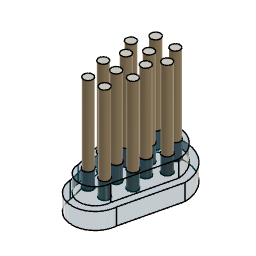
Molde Interior (Autodesk Fusion 360 design; units mm, degrees)
Autodesk Fusion 360 part; units mm, degrees
sketch "Boceto1" plane through (0, 0, 0) normal (0, 0, 1) x (1, 0, 0)
  line L0 (0, 0) -> (0, 9) construction
  arc A0 (-10, 9) -> (10, 9) centre (0, 10.0556) ccw construction
  line L1 (10, 9) -> (14, 26) construction
  arc A1 (14.9995, 25.882) -> (-14.9995, 25.882) centre (0, 26) ccw construction
  line L2 (-10, 9) -> (-14, 26) construction
  line L3 (-10, 9) -> (10, 9) construction
  line L4 (0, 40) -> (0, 26) construction
  arc A2 (-10.9875, 8.8309) -> (10.9875, 8.8309) centre (0, 10.0556) ccw construction
  line L5 (10.9875, 8.8309) -> (14.9995, 25.882) construction
  line L6 (-10.9875, 8.8309) -> (-14.9995, 25.882) construction
  arc A3 (14, 26) -> (-14, 26) centre (0, 26) ccw construction
  line L7 (-14, 26) -> (14, 26) construction
  line L8 (0, 0) -> (0, 40) construction
  arc A4 (10.9951, 26.3275) -> (-10.9951, 26.3275) centre (0, 26) ccw
  line L9 (-7.0326, 9.4867) -> (-10.9951, 26.3275)
  arc A5 (-7.0326, 9.4867) -> (7.0326, 9.4867) centre (0, 10.0556) ccw
  line L10 (7.0326, 9.4867) -> (10.9951, 26.3275)
  dimension "d1" = 1
  dimension "d2" = 40
  dimension "d3" = 9
  dimension "d4" = 14
  dimension "d5" = 28
  dimension "d6" = 20
  dimension "d7" = 3
  constraint coincident L0.start L8.start
  constraint vertical L8
  constraint parallel L0 L8
  constraint parallel L4 L8
  constraint perpendicular L4 L7
  constraint midpoint A1.centre L7
  constraint horizontal L3
  constraint midpoint L0.end L3
  constraint coincident L4.start A3
  constraint coincident L0.start A0
  measures "d2" distance of L0.start L4.start
  measures "d3" distance of L0.end L0.start
  measures "d4" distance of L4.start A1.centre
  measures "d5" distance of L1.end L2.end
  measures "d6" distance of A0.start A0.end
extrude "Extruir1" add sketch "Boceto1" along normal blind 5 makes body 1
sketch "Boceto2" plane through (0, 0, 5) normal (0, 0, 1) x (-1, 0, 0)
  arc A0 (7.0326, -9.4867) -> (-7.0326, -9.4867) centre (0, -10.0556) ccw
  line L0 (-7.0326, -9.4867) -> (-10.9951, -26.3275)
  arc A1 (-10.9951, -26.3275) -> (10.9951, -26.3275) centre (0, -26) ccw
  line L1 (10.9951, -26.3275) -> (7.0326, -9.4867)
  line L2 (8.8845, -26.5258) -> (4.949, -9.8)
  arc A2 (4.949, -9.8) -> (-4.949, -9.8) centre (0, -10.0556) ccw
  line L3 (-4.949, -9.8) -> (-8.8845, -26.5258)
  arc A3 (-8.8845, -26.5258) -> (8.8845, -26.5258) centre (0, -26) ccw
  dimension "d10" = -2.1
extrude "Extruir2" add sketch "Boceto2" along normal blind 5 contours L2 A2 L3 A3 bodies 1
sketch "Boceto3" plane through (0, 0, 10) normal (0, 0, 1) x (-1, 0, 0)
  arc A0 (-8.8845, -26.5258) -> (8.8845, -26.5258) centre (0, -26) ccw
  line L0 (8.8845, -26.5258) -> (4.949, -9.8)
  arc A1 (4.949, -9.8) -> (-4.949, -9.8) centre (0, -10.0556) ccw
  line L1 (-4.949, -9.8) -> (-8.8845, -26.5258)
  line L2 (0, -34.9) -> (0, -5.1) construction
  line L3 (0, -20) -> (7.349, -20) construction
  line L4 (0, -20) -> (-7.349, -20) construction
  circle A2 centre (3, -31.4) radius 1.5
  line L5 (0, -34.9) -> (0, -31.4) construction
  line L6 (0, -31.4) -> (3, -31.4) construction
  circle A3 centre (-3, -31.4) radius 1.5
  line L7 (0, -34.9) -> (0, -26.4) construction
  line L8 (0, -26.4) -> (5.5, -26.4) construction
  circle A4 centre (5.5, -26.4) radius 1.5
  circle A5 centre (-5.5, -26.4) radius 1.5
  circle A6 centre (0, -26.4) radius 1.5
  circle A7 centre (3, -22.4) radius 1.5
  circle A8 centre (-3, -22.4) radius 1.5
  circle A9 centre (0, -16.4) radius 1.5
  circle A10 centre (-3, -10.4) radius 1.5 construction
  circle A11 centre (3, -10.4) radius 1.5 construction
  circle A12 centre (5.5, -17) radius 1.5 construction
  circle A13 centre (-5.5, -17) radius 1.5 construction
  line L9 (5.5, -17) -> (4.5, -17) construction
  circle A14 centre (4.5, -17) radius 1.5
  line L10 (-5.5, -17) -> (-4.5, -17) construction
  circle A15 centre (-4.5, -17) radius 1.5
  line L11 (3, -10.4) -> (2.5, -10.4) construction
  line L12 (-3, -10.4) -> (-2.5, -10.4) construction
  circle A16 centre (2.5, -10.4) radius 1.5
  circle A17 centre (-2.5, -10.4) radius 1.5
  dimension "d13" = 3
  dimension "d14" = 3.5
  dimension "d15" = 3
  dimension "d16" = 3
  dimension "d17" = 3
  dimension "d18" = 5
  dimension "d21" = 0
  dimension "d22" = 9
  dimension "d25" = 0
  dimension "d26" = 10
  dimension "d29" = 0
  dimension "d30" = 21
  dimension "d35" = 5.5
  dimension "d38" = 1
  dimension "d39" = 3
  dimension "d40" = 3
  dimension "d41" = 0.5
  dimension "d42" = 0.5
  dimension "d43" = 3
  dimension "d44" = 3
  dimension "d45" = 1
  constraint midpoint A0 L2.start
  constraint midpoint A1 L2.end
  constraint midpoint L2 L3.start
  constraint coincident L0 L3.end
  constraint perpendicular L2 L3
  constraint coincident L1 L4.end
  constraint perpendicular L2 L4
  constraint parallel L2 L5
  constraint perpendicular L5 L6
  constraint symmetric L2 A2 A3
  constraint coincident L2 L7.end
  constraint parallel L2 L7
  constraint perpendicular L7 L8
  constraint coincident L8.end A4.centre
  constraint symmetric L2 A4 A5
  constraint coincident L7.end L8.start
  constraint coincident A2.centre L6.end
  constraint coincident A12.centre L9.start
  constraint perpendicular L2 L9
  constraint coincident L9.end A14.centre
  constraint coincident A13.centre L10.start
  constraint horizontal L10
  constraint coincident L10.end A15.centre
  constraint coincident A11.centre L11.start
  constraint perpendicular L2 L11
  constraint coincident A10.centre L12.start
  constraint horizontal L12
  constraint coincident L11.end A16.centre
  constraint coincident L12.end A17.centre
  measures "d13" diameter of A2
  measures "d14" distance of L2.start L5.end
  measures "d15" distance of L5.end A2.centre
  measures "d16" diameter of A4
  measures "d17" diameter of A6
  measures "d18" distance of L5.end L7.end
  measures "d35" distance of L7.end L8.end
  measures "d38" distance of A12.centre L9.end
  measures "d39" diameter of A14
  measures "d40" diameter of A15
  measures "d41" distance of A10.centre L12.end
  measures "d42" distance of A11.centre L11.end
  measures "d43" diameter of A16
  measures "d44" diameter of A17
  measures "d45" distance of A13.centre L10.end
extrude "Extruir3" add sketch "Boceto3" along normal blind 24 separate body contours A2 | A3 | A4 | A5 | A6 | A7 | A8 | A9 | A14 | A15 | A16 | A17 makes body 2 at (3.0019, 17.0748, 26) makes body 3 at (4.0019, 26.4748, 26) makes body 4 at (1.5019, 22.4748, 26) makes body 5 at (-4.4981, 22.4748, 26) makes body 6 at (4.4095, 31.913, 26) makes body 7 at (-3.9981, 10.4748, 26) makes body 8 at (-5.9981, 17.0748, 26) makes body 9 at (-6.9981, 26.4748, 26) makes body 10 at (-1.4981, 16.4748, 26) makes body 11 at (-1.4981, 26.4748, 26) makes body 12 at (-1.5905, 31.913, 26) makes body 13 at (1.0019, 10.4748, 26)
extrude "Extruir4" cut sketch "Boceto3" against normal blind 5 contours A2 | A3 | A4 | A5 | A6 | A7 | A8 | A9 | A14 | A15 | A16 | A17 bodies 1
extrude "Extruir5" add 12 faces at (-2.084, 10.2947, 10) (-2.75, 23.2669, 10) (-4.2334, 15.9775, 10) (-0.4671, 16.6898, 10) (2.6931, 10.7148, 10) (4.0495, 16.9321, 10) (3.25, 23.2669, 10) (0.25, 27.2669, 10) (-5.9944, 27.1547, 10) (-2.7722, 31.9804, 10) (3.1605, 32.0128, 10) (5.0329, 26.6898, 10) along direction (0, 0, -1) blind 5 on bodies 2 3 4 5 6 7 8 9 10 11 12 13 bodies 7 2 3 4 5 6 8 9 10 11 12 13
sketch "Boceto4" plane through (0, 0, 34) normal (0, 0, 1) x (-1, 0, 0)
  circle A0 centre (2.5, -10.4) radius 1.5
  circle A1 centre (-2.5, -10.4) radius 1.5
  circle A2 centre (0, -16.4) radius 1.5
  circle A3 centre (4.5, -17) radius 1.5
  circle A4 centre (-4.5, -17) radius 1.5
  circle A5 centre (-3, -22.4) radius 1.5
  circle A6 centre (3, -22.4) radius 1.5
  circle A7 centre (0, -26.4) radius 1.5
  circle A8 centre (-5.5, -26.4) radius 1.5
  circle A9 centre (-3, -31.4) radius 1.5
  circle A10 centre (3, -31.4) radius 1.5
  circle A11 centre (5.5, -26.4) radius 1.5
  circle A12 centre (4.5, -17) radius 1.5
  circle A13 centre (3, -31.4) radius 1.45
  circle A14 centre (-3, -31.4) radius 1.4
  circle A15 centre (5.5, -26.4) radius 1.4
  circle A16 centre (0, -26.4) radius 1.4
  circle A17 centre (-5.5, -26.4) radius 1.4
  circle A18 centre (3, -22.4) radius 1.4
  circle A19 centre (-3, -22.4) radius 1.4
  circle A20 centre (4.5, -17) radius 1.4
  circle A21 centre (0, -16.4) radius 1.4
  circle A22 centre (-4.5, -17) radius 1.4
  circle A23 centre (2.5, -10.4) radius 1.4
  circle A24 centre (-2.5, -10.4) radius 1.4
  dimension "d50" = 2.9
  dimension "d51" = -0.1
  dimension "d52" = -0.1
  dimension "d53" = -0.1
  dimension "d54" = -0.1
  dimension "d55" = -0.1
  dimension "d56" = -0.1
  dimension "d57" = -0.1
  dimension "d58" = -0.1
  dimension "d59" = -0.1
  dimension "d60" = -0.1
  dimension "d61" = -0.1
  constraint concentric A10 A13
  measures "d50" diameter of A13
extrude "Extruir6" cut sketch "Boceto4" against normal blind 29.5 bodies 2 3 4 5 6 7 8 9 10 11 12 13
